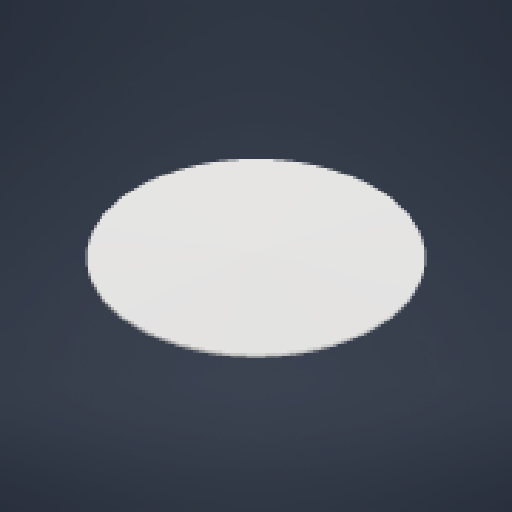
# Autodesk Inventor part: centrer centrifugal spinner
Saved by Autodesk Inventor 2026.1 (Build 301233000, 233)
## iProperties
Created: 2026-03-26
Part Number: centrer centrifugal spinner
Material: Generic
Document SubType Name: Modeling
Designer: sniel
Density: 1 g/cm^3
Appearance: Default
Author: sniel
Autodesk Inventor part; units mm, degrees
ref_plane "YZ Plane" through (0, 0, 0) normal (1, 0, 0) x (0, 1, 0)
ref_plane "XZ Plane" through (0, 0, 0) normal (0, 1, 0) x (-1, 0, 0)
ref_plane "XY Plane" through (0, 0, 0) normal (0, 0, 1) x (1, 0, 0)
sketch "Sketch1" plane through (0, 0, 0) normal (0, 0, 1) x (1, 0, 0)
  line L0 (-98, 0) -> (-98, 2)
  line L1 (-98, 2) -> (0, 5)
  line L2 (0, 5) -> (0, 0)
  line L3 (0, 0) -> (-98, 0)
  line L4 (0, -25) -> (0, 10) projected
  point P0 (0, -20)
  dimension "d3" = 2
  constraints: 8 end point, 2 vertical, 1 perpendicular
  measures "d3" distance of L0.start L0.end
revolve "Revolution1" add sketch "Sketch1" angle 360 about axis through (0, -10, 0) along (0, 1, 0)
sketch "Sketch2" plane through (0, 0, 0) normal (0, -1, 0) x (1, 0, 0)
  circle A0 centre (0, 0) radius 5
  line L0 (-2.5, -15.4211) -> (2.5, -15.4211)
  line L1 (2.5, -15.4211) -> (2.5, 15.4211)
  line L2 (2.5, 15.4211) -> (-2.5, 15.4211)
  line L3 (-2.5, 15.4211) -> (-2.5, -15.4211)
  line L4 (-2.5, -15.4211) -> (2.5, 15.4211) construction
  line L5 (2.5, -15.4211) -> (-2.5, 15.4211) construction
  point P0 (-2.5, 4.3301)
  point P1 (-2.5, -4.3301)
  point P2 (2.5, -4.3301)
  point P3 (2.5, 4.3301)
  dimension "d8" = 10
  dimension "d9" = 5
  constraints: 12 end point, 2 midpoint, 2 parallel, 1 centre point, 1 coincident, 1 horizontal, 1 perpendicular
  measures "d8" diameter of A0
  measures "d9" distance of L2.end L1.end
extrude "Extrusion1" cut sketch "Sketch2" against normal blind 3 contours L1 A0 L3
body "Solid1"
